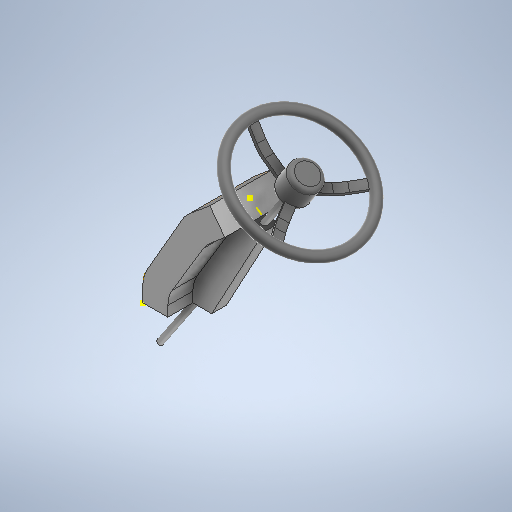
# Autodesk Inventor part: Devarsh_Steering-wheelfinalpart2
Saved by Autodesk Inventor 2025 (Build 290162000, 162)
## iProperties
Created: 2024-10-17
Part Number: Devarsh_Steering-wheelfinalpart2
Material: Generic
Document SubType Name: Modeling
Designer: Hp
Density: 1 g/cm^3
Appearance: Default
Author: Hp
Autodesk Inventor part; units mm, degrees
sketch "Sketch1" plane through (0, 0, 0) normal (0, 0, 1) x (1, 0, 0)
  line L0 (0, 0) -> (0, 53.205081)
  line L1 (13.39746, 103.205081) -> (135.521218, 314.729636)
  line L2 (157.844998, 341.33408) -> (227.760319, 400)
  arc A0 (13.39746, 103.205081) -> (0, 53.205081) centre (100, 53.205081) ccw
  arc A1 (157.844998, 341.33408) -> (135.521218, 314.729636) centre (222.123759, 264.729636) ccw
  line L3 (227.760319, 400) -> (278.841552, 332.061001)
  line L4 (278.841552, 332.061001) -> (227.995952, 289.079724)
  line L5 (206.939042, 264.383733) -> (99.385568, 86.186055)
  line L6 (85, 34.512376) -> (85, 0)
  line L7 (85, 0) -> (0, 0)
  arc A2 (227.995952, 289.079724) -> (206.939042, 264.383733) centre (292.553474, 212.710054) ccw
  arc A3 (99.385568, 86.186055) -> (85, 34.512376) centre (185, 34.512376) ccw
  point P0 (0, 80)
  point P1 (144.337567, 330)
  point P2 (253.418752, 310.570362)
  point P3 (153.162305, 175.284894)
  dimension "d0" = 80
  dimension "d1" = 250
  dimension "d2" = 150
  dimension "d3" = 400
  dimension "d4" = 20
  dimension "d5" = 100
  dimension "d6" = 100
  dimension "d9" = 85
  dimension "d10" = 85
  dimension "d11" = 85
  dimension "d12" = 85
  dimension "d13" = 100
  constraints: 16 end point, 8 point on circle, 8 tangent, 4 centre point, 4 point on line, 2 midpoint, 2 vertical, 1 equal radius, 1 horizontal
  measures "d0" distance of L0.start point (0, 80)
  measures "d1" vertical distance of point (0, 80) point (144.338, 330)
  measures "d2" angle of L0 L1
  measures "d3" vertical distance of L0.start L2.end
  measures "d4" angle of L1 L2
  measures "d5" radius of A0
  measures "d6" radius of A1
  measures "d9" distance of L2.end L3.end
  measures "d10" distance of L6.end L0.start
  measures "d11" distance from line of L2 point (253.419, 310.57)
  measures "d12" distance from line of L1 point (153.162, 175.285)
  measures "d13" radius of A2
surface extrude "ExtrusionSrf1" sketch "Sketch1" along normal mid plane 220 shown yes curves L2 A1 L1 A0 L0
sketch "Sketch2" plane through (13.39746, 103.205081, 110) normal (0.8660254, -0.5, 0) x (0, 0, -1)
  point P0 (110, -96.076952)
extrude "Extrusion1" add sketch "Sketch1" along normal mid plane 220
sketch "Sketch3" plane through (0, 0, 0) normal (0, 0, 1) x (1, 0, 0)
  line L0 (85, 0) -> (149.345579, 0)
  line L1 (149.345579, 0) -> (328.841552, 332.061001)
  line L2 (227.995952, 289.079724) -> (278.841552, 332.061001)
  line L3 (328.841552, 332.061001) -> (278.841552, 332.061001)
  line L4 (278.841552, 332.061001) -> (227.995952, 289.079724)
  arc A0 (227.995952, 289.079724) -> (199.973259, 252.842624) centre (298.674137, 205.469488) ccw
  arc A1 (99.385568, 86.186055) -> (85, 34.512376) centre (185, 34.512376) ccw
  line L5 (199.973259, 252.842624) -> (99.385568, 86.186055)
  line L6 (85, 0) -> (85, 34.512376)
  line L7 (99.385568, 86.186055) -> (210.766994, 270.725994)
  point P0 (0, 0)
  point P1 (199.973259, 252.842624)
  dimension "d16" = 50
  constraints: 14 end point, 4 tangent, 3 point on circle, 1 centre point, 1 collinear, 1 horizontal, 1 parallel, 1 point on line, 1 vertical
  measures "d16" distance of L1.end L2.end
extrude "Extrusion2" add sketch "Sketch3" along normal mid plane 50 contours L6 A1 L5 L7 A0 L2 L3 L1 L0
ref_plane "Work Plane1" through (328.841552, 332.061001, 0) normal (-0.5578313, -0.8299544, 0) x (0, 0, 1)
sketch "Sketch4" plane through (328.841552, 332.061001, 0) normal (-0.5578313, -0.8299544, 0) x (0, 0, 1)
  point P0 (0, 87.689488)
sketch "Sketch5" plane through (328.841552, 332.061001, 0) normal (-0.5578313, -0.8299544, 0) x (0, 0, 1)
  line L0 (-25, -36.260532) -> (-25, 17.143365)
  circle A0 centre (0, 20.649127) radius 10
  point P0 (0, 87.689488)
  dimension "d19" = 20
  constraints: 1 centre point
  measures "d19" diameter of A0
sketch "Sketch6" plane through (328.841552, 332.061001, 0) normal (-0.5578313, -0.8299544, 0) x (0, 0, 1)
  point P0 (0, 87.689488)
extrude "Extrusion3" add sketch "Sketch5" along normal blind 649 and the other way blind 150
sketch "Sketch8" plane through (0, 0, 110) normal (0, 0, 1) x (1, 0, 0)
  point P0 (0, 0)
ref_plane "Work Plane2" through (0, 0, 110) normal (0, 0, 1) x (1, 0, 0)
sketch "Sketch10" plane through (0, 0, 110) normal (0, 0, 1) x (1, 0, 0)
  line L0 (403.67795, 462.494576) -> (387.078862, 473.651201)
  point P0 (0, 0)
sketch "Sketch11" plane through (0, 0, 110) normal (0, 0, 1) x (1, 0, 0)
  point P0 (0, 0)
sketch "Sketch12" plane through (0, 0, 0) normal (0, 0, 1) x (1, 0, 0)
  line L0 (403.67795, 462.494576) -> (387.078862, 473.651201)
  line L1 (395.378406, 468.072889) -> (451.161531, 551.068328)
  line L2 (451.161531, 551.068328) -> (409.663811, 578.959891)
  line L3 (409.663811, 578.959891) -> (353.880686, 495.964451)
  line L4 (353.880686, 495.964451) -> (395.378406, 468.072889)
  circle A0 centre (236.635179, 590.422365) radius 17.5
  point P0 (0, 0)
  dimension "d45" = 35
  dimension "d46" = 100
  dimension "d47" = 50
  dimension "d48" = 200
  constraints: 8 end point, 4 perpendicular, 1 centre point, 1 midpoint
  measures "d45" diameter of A0
  measures "d46" distance of L2.end L3.end
  measures "d47" distance of L1.end L2.end
  measures "d48" distance from line of L1 A0.centre
sketch "Sketch13" plane through (0, 0, 110) normal (0, 0, 1) x (1, 0, 0)
  point P0 (0, 0)
ref_plane "Work Plane3" through (0, 0, 0) normal (0, 0, 1) x (1, 0, 0)
sketch "Sketch14" plane through (0, 0, 110) normal (0, 0, 1) x (1, 0, 0)
  point P0 (0, 0)
sketch "Sketch15" plane through (0, 0, 0) normal (0, 0, 1) x (1, 0, 0)
  point P0 (0, 0)
sketch "Sketch16" plane through (0, 0, 0) normal (0, 0, 1) x (1, 0, 0)
  point P0 (0, 0)
sketch "Sketch17" plane through (0, 0, 0) normal (0, 0, 1) x (1, 0, 0)
  line L0 (403.67795, 462.494576) -> (387.078862, 473.651201)
  line L1 (395.378406, 468.072889) -> (451.161531, 551.068328)
  line L2 (451.161531, 551.068328) -> (409.663811, 578.959891)
  line L3 (409.663811, 578.959891) -> (353.880686, 495.964451)
  line L4 (353.880686, 495.964451) -> (395.378406, 468.072889)
  circle A0 centre (259.353448, 624.223138) radius 17.5
  line L5 (278.841552, 332.061001) -> (227.760319, 400)
  point P0 (0, 0)
  dimension "d50" = 100
  dimension "d51" = 50
  dimension "d52" = 35
  dimension "d53" = 200
  dimension "d54" = 160
  constraints: 8 end point, 3 perpendicular, 1 centre point, 1 midpoint
  measures "d50" distance of L1.start L1.end
  measures "d51" distance of L1.end L2.end
  measures "d52" diameter of A0
  measures "d53" distance from line of L1 A0.centre
  measures "d54" distance from line of L5 A0.centre
sketch "Sketch18" plane through (0, 0, 110) normal (0, 0, 1) x (1, 0, 0)
  point P0 (0, 0)
sketch "Sketch19" plane through (0, 0, 110) normal (0, 0, 1) x (1, 0, 0)
  point P0 (0, 0)
ref_plane "Work Plane4" through (0, 0, 0) normal (0, 0, 1) x (1, 0, 0)
revolve "Revolution2" add sketch "Sketch17" angle 360 about axis through (395.378406, 468.072889, 0) along (0.5578313, 0.8299544, 0)
sketch "Sketch20" plane through (0, 0, 0) normal (0, 0, 1) x (1, 0, 0)
  point P0 (0, 0)
sketch "Sketch21" plane through (0, 0, 0) normal (0, 0, 1) x (1, 0, 0)
  line L0 (367.824624, 500.000311) -> (319.183865, 534.603806)
  line L1 (291.992792, 563.66798) -> (253.979888, 625.422483)
  line L2 (253.979888, 625.422483) -> (263.175625, 631.082906)
  line L3 (263.175625, 631.082906) -> (298.790801, 573.223672)
  line L4 (325.981874, 544.159498) -> (374.622634, 509.556003)
  line L5 (374.622634, 509.556003) -> (367.824624, 500.000311)
  arc A0 (291.992792, 563.66798) -> (319.183865, 534.603806) centre (377.152386, 616.087857) ccw
  arc A1 (298.790801, 573.223672) -> (325.981874, 544.159498) centre (383.950395, 625.643549) ccw
  point P0 (0, 0)
  point P1 (302.637384, 546.375128)
  point P2 (309.435393, 555.93082)
  dimension "d56" = 80
  dimension "d57" = 80
  dimension "d58" = 100
  dimension "d59" = 100
  constraints: 12 end point, 4 point on circle, 4 point on line, 4 tangent, 3 perpendicular, 2 centre point
  measures "d56" distance of L0.start point (302.637, 546.375)
  measures "d57" distance of point (309.435, 555.931) L4.end
  measures "d58" radius of A0
  measures "d59" radius of A1
extrude "Extrusion5" add sketch "Sketch21" along normal blind 20 and the other way blind 10
pattern_circular "Circular Pattern2" count 3 over 360 about axis through (423.269968, 509.570608, 0) along (0.5578313, 0.8299544, 0) of "Extrusion5"
fillet "Fillet2" radius 15 1 edges at (492.6593, 523.1768, 0)
fillet "Fillet3" radius 15 1 edges at (436.8761, 440.1813, 0)
body "Solid1"
body "Srf1"
